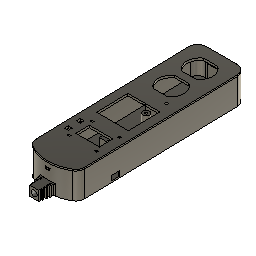
RelaySwitchBox (Autodesk Fusion 360 design; units mm, degrees)
Autodesk Fusion 360 part; units mm, degrees
sketch "Sketch1" plane through (0, 0, 0) normal (0, 1, 0) x (1, 0, 0) in component "Base"
  line L0 (-214.641, -30) -> (-10, -30)
  line L1 (0, -20) -> (0, 20)
  line L2 (-10, 30) -> (-214.641, 30)
  line L3 (0, 0) -> (-211.3181, 0) construction
  line L4 (-230, 30) -> (-230, -30) construction
  arc A0 (-223.3013, 25) -> (-223.3013, -25) centre (-180, 0) ccw
  line L5 (-220, 30) -> (-220, -30) construction
  arc A1 (0, 20) -> (-10, 30) centre (-10, 20) ccw
  arc A2 (-10, -30) -> (0, -20) centre (-10, -20) ccw
  arc A3 (-214.641, 30) -> (-223.3013, 25) centre (-214.641, 20) ccw
  arc A4 (-223.3013, -25) -> (-214.641, -30) centre (-214.641, -20) ccw
  line L6 (-214.641, -32) -> (-10, -32)
  arc A5 (-10, -32) -> (2, -20) centre (-10, -20) ccw
  line L7 (2, -20) -> (2, 20)
  arc A6 (2, 20) -> (-10, 32) centre (-10, 20) ccw
  line L8 (-10, 32) -> (-214.641, 32)
  arc A7 (-214.641, 32) -> (-225.0333, 26) centre (-214.641, 20) ccw
  arc A8 (-225.0333, 26) -> (-225.0333, -26) centre (-180, 0) ccw
  arc A9 (-225.0333, -26) -> (-214.641, -32) centre (-214.641, -20) ccw
  circle A10 centre (-88.5, 0) radius 1.55
  circle A11 centre (-5, 0) radius 1.55
  circle A12 centre (-148, 0) radius 1.55
  circle A13 centre (-148, 0) radius 4.5
  circle A14 centre (-99.5, 0) radius 1.55
  circle A15 centre (-99.5, 0) radius 4.5
  circle A16 centre (-132, -12) radius 5
  line L9 (-232, 0) -> (-232, -49.4784) construction
  line L10 (0, -7.5) -> (-10, -7.5)
  line L11 (-10, -7.5) -> (-10, 7.5)
  line L12 (-10, 7.5) -> (0, 7.5)
  line L13 (0, 7.5) -> (0, -7.5)
  line L14 (0, -7.5) -> (-10, 7.5) construction
  line L15 (-10, -7.5) -> (0, 7.5) construction
  line L16 (-83.5, -7.5) -> (-93.5, -7.5)
  line L17 (-93.5, -7.5) -> (-93.5, 7.5)
  line L18 (-93.5, 7.5) -> (-83.5, 7.5)
  line L19 (-83.5, 7.5) -> (-83.5, -7.5)
  line L20 (-83.5, -7.5) -> (-93.5, 7.5) construction
  line L21 (-93.5, -7.5) -> (-83.5, 7.5) construction
  line L22 (-95, 0) -> (-95, -15.2625) construction
  line L23 (-160.75, 26.5) -> (-185.75, 26.5) construction
  line L24 (-185.75, 26.5) -> (-185.75, -26.5) construction
  line L25 (-185.75, -26.5) -> (-160.75, -26.5) construction
  line L26 (-160.75, -26.5) -> (-160.75, 26.5) construction
  line L27 (-160.75, 26.5) -> (-185.75, -26.5) construction
  line L28 (-185.75, 26.5) -> (-160.75, -26.5) construction
  line L29 (-99.5, 0) -> (-148, 0) construction
  line L30 (-88.5, 0) -> (-5, 0) construction
  line L31 (-94.75, 22.5) -> (-152.75, 22.5) construction
  line L32 (-152.75, 22.5) -> (-152.75, -22.5) construction
  line L33 (-152.75, -22.5) -> (-94.75, -22.5) construction
  line L34 (-94.75, -22.5) -> (-94.75, 22.5) construction
  line L35 (-94.75, 22.5) -> (-152.75, -22.5) construction
  line L36 (-152.75, 22.5) -> (-94.75, -22.5) construction
  line L37 (-11.75, 20) -> (-81.75, 20) construction
  line L38 (-81.75, 20) -> (-81.75, -20) construction
  line L39 (-81.75, -20) -> (-11.75, -20) construction
  line L40 (-11.75, -20) -> (-11.75, 20) construction
  line L41 (-11.75, 20) -> (-81.75, -20) construction
  line L42 (-81.75, 20) -> (-11.75, -20) construction
  line L43 (-99.5, 4.5) -> (-93.5, 4.5)
  line L44 (-99.5, -4.5) -> (-93.5, -4.5)
  line L45 (-148, 4.5) -> (-158, 4.5)
  line L46 (-148, -4.5) -> (-158, -4.5)
  line L47 (-158, -4.5) -> (-158, 4.5)
  point P0 (-5, 0)
  point P1 (-88.5, 0)
  point P2 (-173.25, 0)
  point P3 (-123.75, 0)
  point P4 (-46.75, 0)
  dimension "InteriorWidth" = 60
  dimension "d2" = 10
  dimension "InteriorLength" = 230
  dimension "d4" = 10
  dimension "d5" = 10
  dimension "d6" = 2
  dimension "d11" = 83.5
  dimension "d12" = 3.1
  dimension "d20" = 48.5
  dimension "d22" = 3.1
  dimension "d23" = 9
  dimension "d25" = 10
  dimension "d41" = 10
  dimension "d42" = 15
  dimension "d72" = 53
  dimension "d73" = 25
  dimension "d74" = 58
  dimension "d75" = 45
  dimension "d76" = 70
  dimension "d77" = 40
  dimension "d78" = 11
  dimension "d79" = 8
  dimension "d157" = 10
  dimension "d158" = 2.75
  dimension "d163" = 16
  dimension "d164" = 12
  constraint horizontal L0
  constraint perpendicular L0 L1
  constraint perpendicular L1 L2
  constraint vertical L5.end L5.start
  constraint coincident L3.start origin
  constraint horizontal L3
  constraint symmetric L5.end L5.start L3
  constraint coincident L3.start L1
  constraint coincident L2 L4.start
  constraint coincident L0 L4.end
  constraint perpendicular L0 L4
  constraint tangent L4 A0
  constraint tangent L1 A1
  constraint tangent L2 A1
  constraint tangent L0 A2
  constraint tangent L1 A2
  constraint equal A1 A2
  constraint coincident L5.start L2
  constraint coincident L5.start A0
  constraint tangent L2 A3
  constraint tangent A0 A3
  constraint coincident L5.end L0
  constraint coincident L5.end A0
  constraint tangent L0 A4
  constraint tangent A0 A4
  constraint equal A3 A4
  constraint coincident L3 P1
  constraint coincident L3 P0
  constraint equal A10 A11
  constraint coincident L3 A12.centre
  constraint concentric A12 A13
  constraint coincident L3 A14.centre
  constraint concentric A14 A15
  constraint equal A12 A14
  constraint equal A13 A15
  constraint midpoint A8 L9.start
  constraint tangent A8 L9
  constraint perpendicular L3 L9
  constraint horizontal L10
  constraint perpendicular L10 L11
  constraint parallel L10 L12
  constraint parallel L11 L13
  constraint coincident L1 L10.start
  constraint coincident L14 P0
  constraint coincident L15 P0
  constraint coincident P0 A11.centre
  constraint horizontal L16
  constraint perpendicular L16 L17
  constraint parallel L16 L18
  constraint parallel L17 L19
  constraint coincident L20 P1
  constraint coincident L21 P1
  constraint coincident P1 A10.centre
  constraint equal L11 L19
  constraint equal L12 L18
  constraint coincident L3 L22.start
  constraint coincident A15 L22.start
  constraint tangent A15 L22
  constraint horizontal L23
  constraint perpendicular L23 L24
  constraint parallel L23 L25
  constraint parallel L24 L26
  constraint coincident L27 P2
  constraint coincident L28 P2
  constraint coincident L3 P2
  constraint coincident A14.centre A15.centre
  constraint coincident A12.centre A13.centre
  constraint horizontal L31
  constraint perpendicular L31 L32
  constraint parallel L31 L33
  constraint parallel L32 L34
  constraint coincident L35 P3
  constraint coincident L36 P3
  constraint midpoint L29 P3
  constraint horizontal L37
  constraint perpendicular L37 L38
  constraint parallel L37 L39
  constraint parallel L38 L40
  constraint coincident L41 P4
  constraint coincident L42 P4
  constraint midpoint L30 P4
  constraint coincident A15 L43.start
  constraint coincident L17 L43.end
  constraint tangent A15 L43
  constraint perpendicular L17 L43
  constraint coincident A15 L44.start
  constraint coincident L17 L44.end
  constraint tangent A15 L44
  constraint perpendicular L17 L44
  constraint coincident A13 L45.start
  constraint tangent A13 L45
  constraint perpendicular L32 L45
  constraint coincident A13 L46.start
  constraint tangent A13 L46
  constraint parallel L45 L46
  constraint perpendicular L45 L47
  measures "InteriorWidth" distance of L0 L2
  measures "d2" distance of L4 L5
  measures "InteriorLength" distance of L1 L4
  measures "d4" radius of A1
  measures "d5" radius of A3
  measures "d11" distance of P1 P0
  measures "d12" diameter of A10
  measures "d20" distance of A12.centre A14.centre
  measures "d22" diameter of A14
  measures "d23" diameter of A15
  measures "d25" diameter of A16
  measures "d41" distance of L1 L11
  measures "d42" distance of L10 L12
  measures "d72" distance of L23.start L25.end
  measures "d73" distance of L23.start L23.end
  measures "d74" distance of L32.end L33.end
  measures "d75" distance of L31.start L33.end
  measures "d76" distance of L38.end L39.end
  measures "d77" distance of L37.end L38.end
  measures "d78" distance of P1 A14.centre
  measures "d79" distance of L26 L32
  measures "d157" distance of L46.start L46.end
  measures "d158" distance of L26 L45.end
  measures "d163" horizontal distance of A12.centre A16.centre
  measures "d164" distance of A16.centre L29
extrude "Extrude1" add sketch "Sketch1" along normal blind 2 contours L0 L1 L2 A0 A1 A2 A3 A4 L10 L11 L12 | L1 L10 L11 L12 L13 | L6 A5 L7 A6 L8 A7 A8 A9 | A10 | A11 | A12 | A13 | A13 L45 L46 L47 | A14 | A15 | A15 L17 L43 L44 | L16 L17 L18 L19 makes body 1 in component "Base"
extrude "Extrude2" add sketch "Sketch1" against normal blind 33 contours L6 A5 L7 A6 L8 A7 A8 A9 bodies 1 in component "Base"
extrude "Extrude3" add sketch "Sketch1" against normal blind 21 contours A13 | A13 L45 L46 L47 | A15 bodies 1 in component "Base"
extrude "Extrude4" add sketch "Sketch1" against normal blind 28 contours L1 L10 L11 L12 L13 | L16 L17 L18 L19 bodies 1 in component "Base"
sketch "Sketch1 (2)" plane through (0, 0, 0) normal (0, 1, 0) x (1, 0, 0) in component "CordPlug"
  line L0 (-230, 30) -> (-230, -30)
  line L1 (-232, 0) -> (-232, -49.4784)
  line L2 (-232, 0) -> (-232, -10)
  line L3 (-232, -10) -> (-234, -10)
  line L4 (-234, -10) -> (-234, -5.75)
  line L5 (-234, -5.75) -> (-236, -5.75)
  line L6 (-236, -5.75) -> (-236, -9)
  line L7 (-236, -9) -> (-238, -9)
  line L8 (-238, -9) -> (-238, -5.75)
  line L9 (-238, -5.75) -> (-240, -5.75)
  line L10 (-240, -5.75) -> (-240, -8)
  line L11 (-240, -8) -> (-242, -8)
  line L12 (-242, -8) -> (-242, -5.75)
  line L13 (-242, -5.75) -> (-244, -5.75)
  line L14 (-244, -5.75) -> (-244, -7)
  line L15 (-244, -7) -> (-246, -7)
  line L16 (-246, -7) -> (-246, -5.75)
  line L17 (-246, -5.75) -> (-248, -5.75)
  line L18 (-248, -5.75) -> (-248, -6)
  line L19 (-248, -6) -> (-250, -6)
  line L20 (-250, -6) -> (-250, 0)
  line L21 (0, 0) -> (-211.3181, 0)
  line L22 (-211.3181, 0) -> (-211.3181, -3.75) construction
  line L23 (-211.3181, -3.75) -> (-211.3181, -2.7422) construction
  line L24 (-211.3181, 0) -> (-211.3181, -3.75) construction
  arc A0 (-225.0333, 26) -> (-225.0333, -26) centre (-180, 0) ccw construction
  line L25 (-232, -10) -> (-231.0294, -10)
  line L26 (-232, 0) -> (-248.7319, 0) construction
  line L27 (-232, 0) -> (-232, 10)
  line L28 (-232, 10) -> (-234, 10)
  line L29 (-234, 10) -> (-234, 5.75)
  line L30 (-234, 5.75) -> (-236, 5.75)
  line L31 (-236, 5.75) -> (-236, 9)
  line L32 (-236, 9) -> (-238, 9)
  line L33 (-238, 9) -> (-238, 5.75)
  line L34 (-238, 5.75) -> (-240, 5.75)
  line L35 (-240, 5.75) -> (-240, 8)
  line L36 (-240, 8) -> (-242, 8)
  line L37 (-242, 8) -> (-242, 5.75)
  line L38 (-242, 5.75) -> (-244, 5.75)
  line L39 (-244, 5.75) -> (-244, 7)
  line L40 (-244, 7) -> (-246, 7)
  line L41 (-246, 7) -> (-246, 5.75)
  line L42 (-246, 5.75) -> (-248, 5.75)
  line L43 (-248, 5.75) -> (-248, 6)
  line L44 (-248, 6) -> (-250, 6)
  line L45 (-250, 6) -> (-250, 0)
  line L46 (-232, 10) -> (-231.0294, 10)
  arc A1 (-225.0333, 26) -> (-225.0333, -26) centre (-180, 0) ccw
  line L47 (-232, -5.25) -> (-229.7236, -5.25)
  line L48 (-229.7236, -5.25) -> (-229.7236, -7.25)
  line L49 (-229.7236, -7.25) -> (-227.7236, -7.25)
  line L50 (-227.7236, -7.25) -> (-227.7236, 0)
  line L51 (-232, 5.25) -> (-229.7236, 5.25)
  line L52 (-229.7236, 5.25) -> (-229.7236, 7.25)
  line L53 (-229.7236, 7.25) -> (-227.7236, 7.25)
  line L54 (-227.7236, 7.25) -> (-227.7236, 0)
  arc A2 (-223.3013, 25) -> (-223.3013, -25) centre (-180, 0) ccw
  dimension "d52" = 2
  dimension "d53" = 2
  dimension "d54" = 10
  dimension "d56" = 1
  dimension "d57" = 1
  dimension "d58" = 1
  dimension "d59" = 1
  dimension "d60" = 3.75
  dimension "d61" = 2
  dimension "d69" = 1.5
  dimension "d70" = 2
  dimension "d71" = 2
  constraint coincident L1.start L2.start
  constraint coincident L1 L2.end
  constraint perpendicular L1 L3
  constraint perpendicular L3 L4
  constraint perpendicular L4 L5
  constraint perpendicular L5 L6
  constraint perpendicular L6 L7
  constraint perpendicular L7 L8
  constraint perpendicular L8 L9
  constraint perpendicular L7 L10
  constraint perpendicular L10 L11
  constraint perpendicular L11 L12
  constraint perpendicular L12 L13
  constraint perpendicular L13 L14
  constraint perpendicular L14 L15
  constraint perpendicular L15 L16
  constraint perpendicular L14 L17
  constraint perpendicular L15 L18
  constraint perpendicular L18 L19
  constraint perpendicular L15 L20
  constraint equal L3 L7
  constraint equal L7 L11
  constraint equal L11 L15
  constraint equal L15 L19
  constraint equal L13 L17
  constraint equal L9 L13
  constraint equal L5 L9
  constraint horizontal L1.start L20.end
  constraint horizontal L12.end L16.end
  constraint horizontal L8.end L12.end
  constraint horizontal L4.end L8.end
  constraint coincident L21.end L22.start
  constraint perpendicular L21 L22
  constraint coincident L22 L23.end
  constraint perpendicular L21 L24
  constraint coincident A0 L25.end
  constraint perpendicular L1 L25
  constraint perpendicular L2 L26
  constraint symmetric L1.start L26 L2.start
  constraint symmetric L2.end L26 L27.end
  constraint symmetric L3.end L26 L28.end
  constraint symmetric L4.end L26 L29.end
  constraint symmetric L5.end L26 L30.end
  constraint symmetric L6.end L26 L31.end
  constraint symmetric L7.end L26 L32.end
  constraint symmetric L8.end L26 L33.end
  constraint symmetric L9.end L26 L34.end
  constraint symmetric L10.end L26 L35.end
  constraint symmetric L11.end L26 L36.end
  constraint symmetric L12.end L26 L37.end
  constraint symmetric L13.end L26 L38.end
  constraint symmetric L14.end L26 L39.end
  constraint symmetric L15.end L26 L40.end
  constraint symmetric L16.end L26 L41.end
  constraint symmetric L17.end L26 L42.end
  constraint symmetric L18.end L26 L43.end
  constraint symmetric L19.end L26 L44.end
  constraint symmetric L20.end L26 L45.end
  constraint symmetric L25.end L26 L46.end
  constraint coincident L1 L47.start
  constraint perpendicular L1 L47
  constraint perpendicular L47 L48
  constraint perpendicular L48 L49
  constraint coincident L21 L50.end
  constraint perpendicular L21 L50
  constraint symmetric L26 L47.start L51.start
  constraint symmetric L26 L47.end L51.end
  constraint symmetric L26 L48.end L52.end
  constraint symmetric L26 L49.end L53.end
  constraint symmetric L26 L50.end L54.end
  constraint coincident L47.end A2
  measures "d52" distance of L2.end L3.end
  measures "d53" distance of L4.end L5.end
  measures "d54" distance of L1.start L2.end
  measures "d56" vertical distance of L3.end L6.end
  measures "d57" vertical distance of L7.end L10.end
  measures "d58" vertical distance of L11.end L14.end
  measures "d59" vertical distance of L15.end L18.end
  measures "d60" distance of L21.end L22.end
  measures "d61" vertical distance of L9.end L22.end
  measures "d69" distance of L22.end L47
  measures "d70" distance of L47.end L48.end
  measures "d71" distance of L48.end L49.end
extrude "Extrude1'" add sketch "Sketch1 (2)" against normal blind 13 separate body contours L0 L51 A2 | L0 A1 L47 L51 | L27 L46 A1 L51 | L0 L47 A2 | L49 L50 L53 L54 A2 | L27 A1 L51 | L52 L53 A2 | L1 L2 L3 L4 L5 L6 L7 L8 L9 L10 L11 L12 L13 L14 L15 L16 L17 L18 L19 L20 L27 L28 L29 L30 L31 L32 L33 L34 L35 L36 L37 L38 L39 L40 L41 L42 L43 L44 L45 | L48 L49 A2 | L1 L2 A1 L47 | L1 L2 L25 A1 L47 makes body 2 in component "CordPlug"
sketch "Sketch2" plane through (-250, 0, 0) normal (-1, 0, 0) x (0, 0, 1) in component "CordPlug"
  line L0 (6, 0) -> (-6, 0)
  line L1 (-6, 0) -> (-6, -13)
  line L2 (-6, -13) -> (6, -13)
  line L3 (6, -13) -> (6, 0)
  line L4 (6, -6.5) -> (-6, -6.5) construction
  line L5 (0, 0) -> (0, -13) construction
  circle A0 centre (0, -6.5) radius 3.75
  dimension "d64" = 7.5
  constraint midpoint L3 L4.start
  constraint midpoint L1 L4.end
  constraint coincident L5.start origin
  constraint midpoint L2 L5.end
  constraint midpoint L5 A0.centre
  measures "d64" diameter of A0
extrude "Extrude5" [suppressed] in component "Base"
extrude "Extrude2'" cut sketch "Sketch2" against normal blind 41.205 contours A0 bodies 2 in component "CordPlug"
extrude "Extrude6" add sketch "Sketch1" against normal blind 10 contours A15 L17 L43 L44 bodies 1 in component "Base"
fillet "Fillet1" radius 3 6 edges at (-5, 0, 7.5) (-10, 0, 0) (-5, 0, -7.5) (-83.5, 0, 0) (-88.5, 0, -7.5) (-88.5, 0, 7.5) on bodies 1 in component "Base"
fillet "Fillet1" radius 3 1 edges at (-158, 0, 0) on bodies 1 in component "Base"
sketch "Sketch1 (3)" plane through (0, -33, 0) normal (0, -1, 0) x (1, 0, 0) in component "Lid"
  arc A0 (-10, -30) -> (0, -20) centre (-10, -20) ccw
  line L0 (-10, -30) -> (-214.641, -30)
  arc A1 (-223.3013, -25) -> (-214.641, -30) centre (-214.641, -20) ccw
  arc A2 (-223.3013, 25) -> (-223.3013, -25) centre (-180, 0) ccw
  arc A3 (-214.641, 30) -> (-223.3013, 25) centre (-214.641, 20) ccw
  line L1 (-214.641, 30) -> (-10, 30)
  arc A4 (0, 20) -> (-10, 30) centre (-10, 20) ccw
  line L2 (0, 20) -> (0, -20)
  arc A5 (-214.641, 32) -> (-225.0333, 26) centre (-214.641, 20) ccw
  arc A6 (-225.0333, 26) -> (-225.0333, -26) centre (-180, 0) ccw
  arc A7 (-225.0333, -26) -> (-214.641, -32) centre (-214.641, -20) ccw
  line L3 (-214.641, -32) -> (-10, -32)
  arc A8 (-10, -32) -> (2, -20) centre (-10, -20) ccw
  line L4 (2, -20) -> (2, 20)
  arc A9 (2, 20) -> (-10, 32) centre (-10, 20) ccw
  line L5 (-10, 32) -> (-214.641, 32)
  arc A10 (-223.3013, 25) -> (-223.3013, -25) centre (-180, 0) ccw
  arc A11 (-214.641, 30) -> (-223.3013, 25) centre (-214.641, 20) ccw
  line L6 (-214.641, 30) -> (-10, 30)
  arc A12 (0, 20) -> (-10, 30) centre (-10, 20) ccw
  line L7 (0, 20) -> (0, -20)
  arc A13 (-10, -30) -> (0, -20) centre (-10, -20) ccw
  arc A14 (-223.3013, -25) -> (-214.641, -30) centre (-214.641, -20) ccw
  line L8 (-10, -30) -> (-214.641, -30)
  arc A15 (-225.0333, 26) -> (-225.0333, -26) centre (-180, 0) ccw
  arc A16 (-214.641, 32) -> (-225.0333, 26) centre (-214.641, 20) ccw
  line L9 (-214.641, 32) -> (-10, 32)
  arc A17 (2, 20) -> (-10, 32) centre (-10, 20) ccw
  line L10 (2, 20) -> (2, -20)
  arc A18 (-10, -32) -> (2, -20) centre (-10, -20) ccw
  arc A19 (-225.0333, -26) -> (-214.641, -32) centre (-214.641, -20) ccw
  line L11 (-10, -32) -> (-214.641, -32)
  line L12 (-185.75, -26.5) -> (-185.75, 26.5)
  line L13 (-185.75, 26.5) -> (-160.75, 26.5)
  line L14 (-160.75, 26.5) -> (-160.75, -26.5)
  line L15 (-160.75, -26.5) -> (-185.75, -26.5)
  line L16 (0, 0) -> (-267.0293, 0) construction
  line L17 (-52, -16.75) -> (-80, -16.75) construction
  line L18 (-80, -16.75) -> (-80, 16.75) construction
  line L19 (-80, 16.75) -> (-52, 16.75) construction
  line L20 (-52, 16.75) -> (-52, -16.75) construction
  line L21 (-52, -16.75) -> (-80, 16.75) construction
  line L22 (-80, -16.75) -> (-52, 16.75) construction
  line L23 (-13.5, -16.75) -> (-41.5, -16.75) construction
  line L24 (-41.5, -16.75) -> (-41.5, 16.75) construction
  line L25 (-41.5, 16.75) -> (-13.5, 16.75) construction
  line L26 (-13.5, 16.75) -> (-13.5, -16.75) construction
  line L27 (-13.5, -16.75) -> (-41.5, 16.75) construction
  line L28 (-41.5, -16.75) -> (-13.5, 16.75) construction
  line L29 (-46.75, 0) -> (-46.75, 43.389) construction
  line L30 (-52, -9.25) -> (-80, -9.25) construction
  line L31 (-80, -9.25) -> (-80, 9.25) construction
  line L32 (-80, 9.25) -> (-52, 9.25) construction
  line L33 (-52, 9.25) -> (-52, -9.25) construction
  line L34 (-52, -9.25) -> (-80, 9.25) construction
  line L35 (-80, -9.25) -> (-52, 9.25) construction
  line L36 (-80.5, 0) -> (-80.5, 9.25)
  line L37 (-51.5, 0) -> (-51.5, 9.25)
  line L38 (-80, 20.5088) -> (-52, 20.5088) construction
  arc A20 (-51.5, 9.25) -> (-80.5, 9.25) centre (-66, 0) ccw
  line L39 (-80.5, 9.25) -> (-51.5, 9.25) construction
  line L40 (-80, 9.25) -> (-80.5, 9.25) construction
  line L41 (-52, 9.25) -> (-51.5, 9.25) construction
  line L42 (-51.5, 0) -> (-51.5, -9.25)
  arc A21 (-80.5, -9.25) -> (-51.5, -9.25) centre (-66, 0) ccw
  line L43 (-80.5, 0) -> (-80.5, -9.25)
  line L44 (-42, 0) -> (-42, 9.25)
  arc A22 (-13, 9.25) -> (-42, 9.25) centre (-27.5, 0) ccw
  line L45 (-13, 0) -> (-13, 9.25)
  line L46 (-13, 0) -> (-13, -9.25)
  line L47 (-42, 0) -> (-42, -9.25)
  arc A23 (-42, -9.25) -> (-13, -9.25) centre (-27.5, 0) ccw
  line L48 (-182.25, -19.5) -> (-164.25, -19.5)
  line L49 (-164.25, -19.5) -> (-164.25, 11.5)
  line L50 (-164.25, 11.5) -> (-182.25, 11.5)
  line L51 (-182.25, 11.5) -> (-182.25, -19.5)
  line L52 (-183.75, 25) -> (-178.75, 25)
  line L53 (-178.75, 25) -> (-178.75, 20)
  line L54 (-178.75, 20) -> (-183.75, 20)
  line L55 (-183.75, 20) -> (-183.75, 25)
  line L56 (-167.75, 25) -> (-162.75, 25)
  line L57 (-162.75, 25) -> (-162.75, 20)
  line L58 (-162.75, 20) -> (-167.75, 20)
  line L59 (-167.75, 20) -> (-167.75, 25)
  arc A24 (-0.5, 20) -> (-10, 29.5) centre (-10, 20) ccw
  line L60 (-214.641, 29.5) -> (-10, 29.5)
  arc A25 (-214.641, 29.5) -> (-222.8683, 24.75) centre (-214.641, 20) ccw
  arc A26 (-222.8683, 24.75) -> (-222.8683, -24.75) centre (-180, 0) ccw
  arc A27 (-222.8683, -24.75) -> (-214.641, -29.5) centre (-214.641, -20) ccw
  line L61 (-10, -29.5) -> (-214.641, -29.5)
  arc A28 (-10, -29.5) -> (-0.5, -20) centre (-10, -20) ccw
  line L62 (-0.5, 20) -> (-0.5, -20)
  line L63 (-102.75, -21) -> (-144.75, -21)
  line L64 (-144.75, -21) -> (-144.75, 21)
  line L65 (-144.75, 21) -> (-102.75, 21)
  line L66 (-102.75, 21) -> (-102.75, -21)
  line L67 (-102.75, -21) -> (-144.75, 21) construction
  line L68 (-144.75, -21) -> (-102.75, 21) construction
  line L69 (-173.25, 0) -> (-173.25, 34.027) construction
  circle A29 centre (-148, 0) radius 3.5
  circle A30 centre (-99.5, 0) radius 3.5
  circle A31 centre (-88.5, 0) radius 4.5
  circle A32 centre (-5, 0) radius 4.5
  line L70 (-156.75, -20.5) -> (-158.75, -20.5)
  line L71 (-158.75, -20.5) -> (-158.75, -23.5)
  line L72 (-158.75, -23.5) -> (-156.75, -23.5)
  line L73 (-156.75, -23.5) -> (-156.75, -20.5)
  line L74 (-187.75, -20.5) -> (-189.75, -20.5)
  line L75 (-189.75, -20.5) -> (-189.75, -23.5)
  line L76 (-189.75, -23.5) -> (-187.75, -23.5)
  line L77 (-187.75, -23.5) -> (-187.75, -20.5)
  line L78 (-187.75, 15.5) -> (-189.75, 15.5)
  line L79 (-189.75, 15.5) -> (-189.75, 12.5)
  line L80 (-189.75, 12.5) -> (-187.75, 12.5)
  line L81 (-187.75, 12.5) -> (-187.75, 15.5)
  line L82 (-156.75, 15.5) -> (-158.75, 15.5)
  line L83 (-158.75, 15.5) -> (-158.75, 12.5)
  line L84 (-158.75, 12.5) -> (-156.75, 12.5)
  line L85 (-156.75, 12.5) -> (-156.75, 15.5)
  circle A33 centre (-88.5, -16) radius 1.75
  line L86 (-88.5, -16) -> (-88.5, 0) construction
  line L87 (-88.5, -16) -> (-88.5, -32) construction
  point P0 (-5, 0)
  point P1 (-88.5, 0)
  point P2 (-173.25, 0)
  point P3 (-148, 0)
  point P4 (-99.5, 0)
  point P5 (-66, 0)
  point P6 (-27.5, 0)
  point P7 (-46.75, 0)
  point P8 (-66, 0)
  point P9 (-123.75, 0)
  point P10 (-123.75, 0)
  point P11 (-5, 0)
  point P12 (-88.5, 0)
  point P13 (-99.5, 0)
  point P14 (-148, 0)
  dimension "d87" = 28
  dimension "d88" = 33.5
  dimension "d89" = 10.5
  dimension "d90" = 8.75
  dimension "d91" = 18.5
  dimension "d92" = 0.5
  dimension "d93" = 0.5
  dimension "d98" = 42
  dimension "d99" = 18
  dimension "d100" = 31
  dimension "d102" = 5
  dimension "d103" = 5
  dimension "d104" = 1.5
  dimension "d105" = 2
  dimension "d148" = 15
  dimension "d150" = 9
  dimension "d151" = 7
  dimension "d152" = 3
  dimension "d153" = 2
  dimension "d154" = 6
  dimension "d155" = 14
  dimension "d156" = 2
  dimension "d162" = 3.5
  constraint coincident L16.start origin
  constraint perpendicular L7 L16
  constraint horizontal L17
  constraint perpendicular L17 L18
  constraint parallel L17 L19
  constraint parallel L18 L20
  constraint coincident L21 P8
  constraint coincident L22 P8
  constraint coincident L16 P8
  constraint horizontal L23
  constraint perpendicular L23 L24
  constraint parallel L23 L25
  constraint parallel L24 L26
  constraint coincident L27 P6
  constraint coincident L28 P6
  constraint coincident L16 P6
  constraint equal L19 L25
  constraint equal L20 L26
  constraint coincident P7 L29.start
  constraint perpendicular L16 L29
  constraint symmetric L19.end L24.end L29
  constraint horizontal L30
  constraint perpendicular L30 L31
  constraint parallel L30 L32
  constraint parallel L31 L33
  constraint coincident L20 L30.start
  constraint coincident L34 P8
  constraint coincident L35 P8
  constraint coincident P8 P5
  constraint coincident L16 L36.start
  constraint perpendicular L16 L36
  constraint coincident L16 L37.start
  constraint perpendicular L16 L37
  constraint horizontal L36.end L37.end
  constraint coincident L18 L38.start
  constraint coincident L20 L38.end
  constraint perpendicular L20 L38
  constraint coincident L36 A20.end
  constraint perpendicular L36 L40
  constraint coincident L37 A20.start
  constraint perpendicular L37 L41
  constraint equal L40 L41
  constraint symmetric L16 L36.start L43.start
  constraint symmetric L16 L36.end A21.start
  constraint symmetric L16 L37.start L42.start
  constraint symmetric L16 L37.end L42.end
  constraint symmetric L16 A20 A21
  constraint symmetric L29 L36.start L45.start
  constraint symmetric L29 L36.end A22.start
  constraint symmetric L29 L37.start L44.start
  constraint symmetric L29 L37.end L44.end
  constraint symmetric L29 A20 A22
  constraint symmetric L29 L42.end L47.end
  constraint symmetric L29 A21.start L46.end
  constraint symmetric L29 A21 A23
  constraint horizontal L48
  constraint vertical L49
  constraint horizontal L50
  constraint vertical L51
  constraint horizontal L52
  constraint vertical L53
  constraint horizontal L54
  constraint vertical L55
  constraint horizontal L56
  constraint vertical L57
  constraint horizontal L58
  constraint vertical L59
  constraint equal L53 L59
  constraint equal L52 L56
  constraint horizontal L53.end L58.end
  constraint horizontal L63
  constraint perpendicular L63 L64
  constraint parallel L63 L65
  constraint parallel L64 L66
  constraint coincident L67 P10
  constraint coincident L68 P10
  constraint coincident L16 P10
  constraint equal L64 L65
  constraint coincident P10 P9
  constraint coincident P2 L69.start
  constraint perpendicular L5 L69
  constraint symmetric L53.end L58.end L69
  constraint symmetric L49.end L50.end L69
  constraint coincident P14 P3
  constraint coincident P13 P4
  constraint coincident P12 P1
  constraint coincident P11 P0
  constraint equal A31 A32
  constraint equal A29 A30
  constraint horizontal L70
  constraint vertical L71
  constraint horizontal L72
  constraint vertical L73
  constraint horizontal L74
  constraint vertical L75
  constraint horizontal L76
  constraint vertical L77
  constraint horizontal L78
  constraint vertical L79
  constraint horizontal L80
  constraint vertical L81
  constraint horizontal L82
  constraint vertical L83
  constraint horizontal L84
  constraint vertical L85
  constraint equal L81 L85
  constraint equal L73 L81
  constraint equal L73 L77
  constraint equal L70 L82
  constraint equal L70 L74
  constraint equal L74 L80
  constraint symmetric L69 L80.end L83.end
  constraint symmetric L69 L70.end L74.start
  constraint vertical L70.end L83.end
  constraint vertical P12 A33.centre
  constraint coincident A33.centre L86.start
  constraint perpendicular L16 L86
  constraint coincident L11 L87.end
  constraint perpendicular L11 L87
  constraint equal L86 L87
  measures "d87" distance of L18.end L19.end
  measures "d88" distance of L17.end L18.end
  measures "d89" distance of L20 L24
  measures "d91" distance of L30 L32
  measures "d92" distance of L18 L36
  measures "d98" distance of L64.end L65.end
  measures "d99" distance of L48.start L48.end
  measures "d100" distance of L48 L50
  measures "d102" distance of L52.start L52.end
  measures "d103" distance of L52.start L54.end
  measures "d104" distance of L13 L52
  measures "d105" distance of L14 L57
  measures "d148" distance of L13 L50
  measures "d150" diameter of A32
  measures "d151" diameter of A30
  measures "d152" distance of L82.start L84.end
  measures "d153" distance of L83.end L84.end
  measures "d154" distance of L61 L71.end
  measures "d155" distance of L60 L82.end
  measures "d156" distance of L14 L71
  measures "d162" diameter of A33
extrude "Extrude1''" add sketch "Sketch1 (3)" against normal blind 1 separate body contours L12 L13 L14 L15 | A24 L60 A25 A26 A27 L61 A28 L62 makes body 3 in component "Lid"
extrude "Extrude2''" add sketch "Sketch1 (3)" along normal blind 2 contours A0 L0 A1 A2 A3 L1 A4 L2 A10 A11 L6 A12 L7 A13 A14 L8 | A5 A6 A7 L3 A8 L4 A9 L5 A15 A16 L9 A17 L10 A18 A19 L11 | L12 L13 L14 L15 | A32 | A24 L60 A25 A26 A27 L61 A28 L62 | L66 A30 | L64 A29 | A31 picked at (-97.453, -1.1266) picked at (-146.9709, -0.259) bodies 3 in component "Lid"
sketch "Sketch1 (1)" plane through (0, 0, -32) normal (0, 0, -1) x (-1, 0, 0) in component "Base"
  line L0 (214.641, -33) -> (214.641, 2)
  line L1 (214.641, 2) -> (10, 2)
  line L2 (10, 2) -> (10, -33)
  line L3 (10, -33) -> (214.641, -33)
  line L4 (10, 0) -> (214.641, 0)
  line L5 (168, 0) -> (178.5, 0)
  line L6 (178.5, 0) -> (178.5, -6.25)
  line L7 (178.5, -6.25) -> (168, -6.25)
  line L8 (168, -6.25) -> (168, 0)
  line L9 (168, 0) -> (178.5, -6.25) construction
  line L10 (178.5, 0) -> (168, -6.25) construction
  point P0 (185.75, 0)
  point P1 (160.75, 0)
  point P2 (173.25, 0)
  point P3 (173.25, -3.125)
  dimension "d110" = 10.5
  dimension "d113" = 6.25
  constraint horizontal L5
  constraint vertical L6
  constraint horizontal L7
  constraint vertical L8
  constraint midpoint L9 P3
  constraint vertical P2 P3
  constraint coincident L5 P2
  measures "d110" distance of L6.end L7.end
  measures "d113" distance of L5.end L6.end
extrude "Extrude7" cut sketch "Sketch1 (1)" against normal blind 2 contours L4 L5 L6 L7 L8 bodies 1 in component "Base"
sketch "Sketch4" plane through (0, 0, 0) normal (0, 0, 1) x (1, 0, 0) in component "Lid"
  line L0 (-230, -33) -> (-223.3013, -33)
  line L1 (-229.5, -33) -> (-222.8683, -33)
  line L2 (-229.5, -33) -> (-229.5, -27)
  line L3 (-229.5, -27) -> (-232, -27)
  line L4 (-232, -27) -> (-232, -25)
  line L5 (-232, -25) -> (-228.5, -22.3445)
  line L6 (-228.5, -22.3445) -> (-226.5, -22.3445)
  line L7 (-226.5, -22.3445) -> (-226.5, -33)
  line L8 (-232, -35) -> (-225.0333, -35)
  line L9 (-230, -33) -> (-230, -27.5)
  line L10 (-230, -27.5) -> (-232.5, -27.5)
  line L11 (-232.5, -27.5) -> (-232.5, -24.7517)
  line L12 (-232.5, -24.7517) -> (-228.6682, -21.8445)
  line L13 (-228.6682, -21.8445) -> (-226, -21.8445)
  line L14 (-226, -21.8445) -> (-226, -33)
  line L15 (-231, -27.5) -> (-231, -35)
  line L16 (-230, -33) -> (-231, -33)
  dimension "d114" = 6
  dimension "d115" = 2
  dimension "d116" = 3
  dimension "d117" = 2
  dimension "d118" = -0.5
  dimension "d121" = 1
  constraint coincident L1.start L2.start
  constraint perpendicular L1 L2
  constraint perpendicular L2 L3
  constraint perpendicular L2 L6
  constraint coincident L1 L7.end
  constraint perpendicular L1 L7
  constraint perpendicular L3 L4
  constraint vertical L3.end L8.start
  constraint coincident L10 L15.start
  constraint perpendicular L0 L15
  constraint coincident L8 L15.end
  constraint coincident L0.start L9.start
  constraint coincident L15 L16.end
  constraint perpendicular L15 L16
  measures "d114" distance of L1.start L2.end
  measures "d115" distance of L3.end L4.end
  measures "d116" distance of L2 L7
  measures "d117" distance of L5.end L6.end
  measures "d121" distance of L3.end L15
extrude "Extrude3'" add sketch "Sketch4" along normal mid plane 5 contours L0 L1 L2 L3 L4 L5 L6 L7 bodies 3 in component "Lid"
extrude "Extrude8" cut sketch "Sketch4" along normal mid plane 6 bodies 1 in component "Base"
ref_plane "WorkPlane1" through (0, 0, 14) normal (0, 0, 1) x (1, 0, 0) in component "Lid"
sketch "Sketch5" plane through (0, 0, 14) normal (0, 0, 1) x (1, 0, 0) in component "Lid"
  line L0 (-0.5, -33) -> (-0.5, -27)
  line L1 (-1.5, -22.3445) -> (-3.5, -22.3445)
  line L2 (-3.5, -22.3445) -> (-3.5, -33)
  line L3 (-3.5, -33) -> (-0.5, -33)
  line L4 (-0.5, -32) -> (-10, -32)
  line L5 (-226.5, -32) -> (-229.4368, -32)
  line L6 (-229.4368, -32) -> (-229.4368, -33)
  line L7 (-229.4368, -33) -> (-229.5, -33)
  line L8 (-229.5, -33) -> (-229.5, -27)
  line L9 (-229.5, -27) -> (-232, -27)
  line L10 (-232, -27) -> (-232, -25)
  line L11 (-232, -25) -> (-228.5, -22.3445)
  line L12 (-228.5, -22.3445) -> (-226.5, -22.3445)
  line L13 (-226.5, -22.3445) -> (-226.5, -32)
  line L14 (-226.5, -22.3445) -> (20.9262, -22.3445) construction
  line L15 (-232, -25) -> (20.9262, -25) construction
  line L16 (-229.5, -27) -> (21.1765, -27) construction
  line L17 (-0.5, -27) -> (2, -27)
  line L18 (2, -27) -> (2, -25)
  line L19 (2, -25) -> (-1.5, -22.3445)
  line L20 (0, -33.5) -> (0, -27.5)
  line L21 (0, -27.5) -> (2.5, -27.5)
  line L22 (2.5, -27.5) -> (2.5, -24.7517)
  line L23 (2.5, -24.7517) -> (-1.3318, -21.8445)
  line L24 (-1.3318, -21.8445) -> (-4, -21.8445)
  line L25 (-4, -21.8445) -> (-4, -33.5)
  line L26 (-4, -33.5) -> (0, -33.5)
  line L27 (0, -33.5) -> (1, -33.5)
  line L28 (1, -33.5) -> (1, -27.5)
  point P0 (0, -33)
  point P1 (-0.5, -33)
  point P2 (2, -33)
  dimension "d125" = 3
  dimension "d159" = 2
  dimension "d160" = 0.5
  dimension "d161" = 1
  constraint coincident P1 L0.start
  constraint vertical L0
  constraint perpendicular L0 L1
  constraint perpendicular L1 L2
  constraint perpendicular L0 L3
  constraint coincident L12.end L13.start
  constraint perpendicular L13 L14
  constraint coincident L10.end L11.start
  constraint perpendicular L10 L15
  constraint coincident L8.end L9.start
  constraint perpendicular L8 L16
  constraint perpendicular L0 L17
  constraint perpendicular L16 L18
  constraint coincident L16 L17.end
  constraint coincident L15 L18.end
  constraint coincident L1.start L14
  constraint vertical L17.end P2
  constraint perpendicular L20 L27
  constraint coincident L21 L28.end
  constraint perpendicular L21 L28
  measures "d125" distance of L0 L2
  measures "d159" distance of L1.start L1.end
  measures "d161" distance of L18 L28
extrude "Extrude5'" add sketch "Sketch5" along normal mid plane 5 contours L0 L1 L2 L4 L17 L18 L19 bodies 3 in component "Lid"
mirror "Mirror1" about plane through (0, 0, 0) normal (0, 0, 1) of "Extrude5'" in component "Lid"
sketch "Sketch6" plane through (0, 0, 14) normal (0, 0, 1) x (1, 0, 0) in component "Lid"
extrude "Extrude11" cut sketch "Sketch5" along normal mid plane 6 contours L0 L2 L3 L4 | L0 L1 L2 L4 L17 L18 L19 | L20 L21 L22 L23 L24 L25 L26 | L20 L21 L27 L28 bodies 1 in component "Base"
mirror "Mirror2" about plane through (0, 0, 0) normal (0, 0, 1) of "Extrude11" in component "Base"
sketch "Sketch2 (2)" plane through (-227.7236, 0, 0) normal (1, 0, 0) x (0, 0, -1) in component "Base"
  circle A0 centre (0, -6.5) radius 3.75
  line L0 (7.25, 0) -> (-7.25, 0)
  line L1 (-7.25, 0) -> (-7.25, -13)
  line L2 (-7.25, -13) -> (7.25, -13)
  line L3 (7.25, -13) -> (7.25, 0)
  line L4 (5.25, 0) -> (5.25, -13)
  line L5 (-5.25, 0) -> (-5.25, -13)
  point P0 (5.25, 0)
  point P1 (-5.25, 0)
  constraint coincident P0 L4.start
  constraint coincident L2 L4.end
  constraint perpendicular L2 L4
  constraint coincident P1 L5.start
  constraint coincident L2 L5.end
  constraint perpendicular L2 L5
extrude "Extrude12" cut sketch "Sketch2 (2)" against normal blind 49.952 contours A0 | L0 L2 L4 L5 bodies 1 in component "Base"
component "Base" placed x (1, 0, 0) y (0, 1, 0) z (0, 0, 1) at (0, 0, 0)
component "CordPlug" placed x (1, 0, 0) y (0, 1, 0) z (0, 0, 1) at (0, 0, 0)
component "Lid" placed x (1, 0, 0) y (0, 1, 0) z (0, 0, 1) at (0, 0, 0)
equation "d6 = WallThickness"
equation "d12 = 3.35 mm - 0.25 mm"
equation "d46 = -OverallInteriorHeight"
equation "d50 = -( OverallInteriorHeight - 5 mm )"
equation "d57 = d56"
equation "d58 = d56"
equation "d59 = d56"
equation "d60 = ( 7.5 / 2 ) * 1 mm"
equation "WallThickness = 2 mm"
equation "OverallInteriorHeight = 33 mm"
equation "d111 = -WallThickness"
